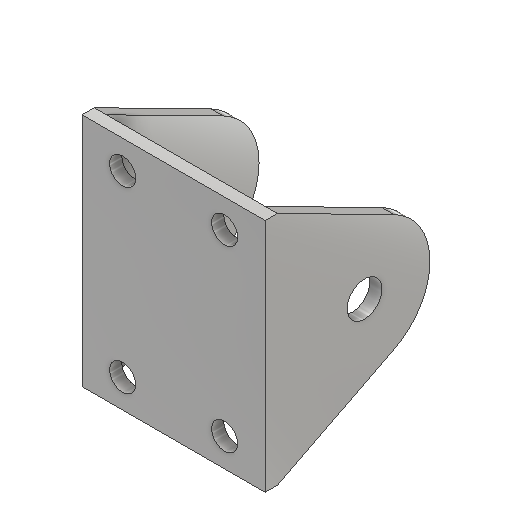
# Autodesk Inventor part: CNCM_Y_Axis_Tensioning_System_C_Sec_Idler
Saved by Autodesk Inventor 2026.1 (Build 301233000, 233)
## iProperties
Created: 2017-08-27
Part Number: CNCM_Y_Axis_Tensioning_System_C_Sec_Idler
Material: Ogólny
Document SubType Name: Modeling
Designer: Andrzej
Density: 1 g/cm^3
Appearance: Aluminium - polerowane
Author: Andrzej
Autodesk Inventor part; units mm, degrees
ref_plane "YZ Plane" through (0, 0, 0) normal (1, 0, 0) x (0, 1, 0)
ref_plane "XZ Plane" through (0, 0, 0) normal (0, 1, 0) x (-1, 0, 0)
ref_plane "XY Plane" through (0, 0, 0) normal (0, 0, 1) x (1, 0, 0)
sketch "Szkic1" plane through (0, 0, 0) normal (0, 0, 1) x (1, 0, 0)
  line L0 (-13.7667, 13.4433) -> (-13.7667, -6.5567)
  line L1 (-13.7667, -6.5567) -> (7.2333, -6.5567)
  line L2 (7.2333, -6.5567) -> (7.2333, 13.4433)
  line L3 (7.2333, 13.4433) -> (5.8333, 13.4433)
  line L4 (-13.7667, 13.4433) -> (-12.3667, 13.4433)
  line L5 (-12.3667, -5.1567) -> (5.8333, -5.1567)
  line L6 (5.8333, -5.1567) -> (5.8333, 13.4433)
  line L7 (-12.3667, 13.4433) -> (-12.3667, -5.1567)
  point P0 (0, 0)
  dimension "d0" = 21
  dimension "d1" = 20
  dimension "d2" = 1.4
  dimension "d3" = 1.4
  dimension "d4" = 1.4
  constraints: 16 end point, 3 perpendicular, 3 vertical, 2 horizontal
  measures "d0" distance of L0.end L1.end
  measures "d1" distance of L0.start L0.end
  measures "d2" distance of L2.end L3.end
  measures "d3" distance of L0.start L4.end
  measures "d4" distance between parallel lines of L1 L5
extrude "Wyciągnięcie proste1" add sketch "Szkic1" along normal blind 27
sketch "Szkic2" plane through (-13.7667, -6.5567, 0) normal (-1, 0, 0) x (0, 0, 1)
  line L0 (0, 20) -> (0, 0) projected
  line L1 (0, 0) -> (27, 0) projected
  line L2 (27, 20) -> (27, 0) projected
  line L3 (0, 20) -> (27, 20) projected
  line L4 (0, 1.4) -> (27, 1.4) projected
  arc A0 (20.1851, 14.7999) -> (6.8149, 14.7999) centre (13.5, 11.4) ccw
  line L5 (27, 1.4) -> (27, 20) projected
  line L6 (27, 1.4) -> (20.1851, 14.7999)
  line L7 (0, 1.4) -> (0, 20) projected
  line L8 (0, 1.4) -> (6.8149, 14.7999)
  line L9 (6.8149, 14.7999) -> (9.4595, 20)
  line L10 (20.1851, 14.7999) -> (17.5405, 20)
  point P0 (0, 6.5567)
  dimension "d7" = 27
  dimension "d8" = 13.5
  dimension "d9" = 10
  dimension "d10" = 15
  constraints: 8 end point, 4 tangent, 2 point on circle, 2 point on line, 1 centre point, 1 coincident
  measures "d7" distance between parallel lines of L0 L2
  measures "d8" distance from line of L2 point (13.5, 11.4)
  measures "d9" distance from line of L4 point (13.5, 11.4)
  measures "d10" diameter of A0
extrude "Wyciągnięcie proste2" cut sketch "Szkic2" against normal through all contours L3 L9 L8 L0 | L3 L10 A0 L9 | L6 L10 L3 L2
hole "Otwór1" at (-13.7667, 4.8433, 13.5) direction (1, 0, 0) diameter 4 end through all
sketch "Szkic3" plane through (-12.3667, -5.1567, 0) normal (0, 1, 0) x (1, 0, 0)
  line L0 (18.2, 0) -> (0, 0) projected
  line L1 (0, 0) -> (0, -27) projected
  line L2 (18.2, -27) -> (0, -27) projected
  line L3 (18.2, 0) -> (18.2, -27) projected
  line L4 (18.2, -20.5) -> (0, -20.5)
  line L5 (18.2, -6.5) -> (0, -6.5)
  point P0 (12.3667, 0)
  point P1 (14.95, -23.75)
  point P2 (3.25, -23.75)
  point P3 (14.95, -3.25)
  point P4 (3.25, -3.25)
  dimension "d20" = 14
  dimension "d21" = 27
  dimension "d22" = 6.5
  dimension "d23" = 3.25
  dimension "d24" = 3.25
  dimension "d25" = 3.25
  dimension "d26" = 3.25
  dimension "d27" = 3.25
  dimension "d28" = 3.25
  dimension "d29" = 3.25
  dimension "d30" = 3.25
  constraints: 4 end point, 4 point on line, 2 perpendicular
  measures "d20" distance between parallel lines of L5 L4
  measures "d21" distance between parallel lines of L0 L2
  measures "d22" distance between parallel lines of L2 L4
  measures "d23" distance from line of L4 point (14.95, -23.75)
  measures "d24" distance from line of L4 point (3.25, -23.75)
  measures "d25" distance from line of L5 point (14.95, -3.25)
  measures "d26" distance from line of L5 point (3.25, -3.25)
  measures "d27" distance from line of L3 point (14.95, -3.25)
  measures "d28" distance from line of L1 point (3.25, -3.25)
  measures "d29" distance from line of L1 point (3.25, -23.75)
  measures "d30" distance from line of L3 point (14.95, -23.75)
hole "Otwór2" at (2.5833, -5.1567, 23.75) at (-9.1167, -5.1567, 23.75) at (2.5833, -5.1567, 3.25) at (-9.1167, -5.1567, 3.25) direction (0, -1, 0) diameter 3 end through all
equation "\"d8\" = 0.5 * d7"
equation "\"d22\" = -0.5 * d20 + 0.5 * d21"
equation "\"d23\" = 0.5 * d22"
equation "\"d24\" = d23"
equation "\"d25\" = d23"
equation "\"d26\" = d23"
equation "\"d27\" = d23"
equation "\"d28\" = d23"
equation "\"d29\" = d23"
equation "\"d30\" = d23"
